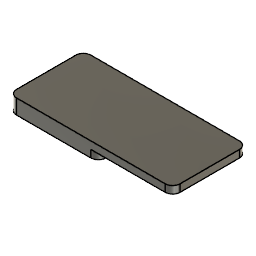
TAPAMESA (Autodesk Fusion 360 design; units mm, degrees)
part number: 2026-05-18-08-57-28-137
Autodesk Fusion 360 part; units mm, degrees
sketch "Sketch4" plane through (0, 0, 0) normal (0, 0, 1) x (1, 0, 0)
  line L0 (50, 0) -> (550, 0)
  line L1 (600, 50) -> (600, 450)
  line L2 (550, 500) -> (50, 500)
  line L3 (0, 450) -> (0, 50)
  arc A0 (600, 450) -> (550, 500) centre (550, 450) ccw
  arc A1 (550, 0) -> (600, 50) centre (550, 50) ccw
  arc A2 (50, 500) -> (0, 450) centre (50, 450) ccw
  arc A3 (0, 50) -> (50, 0) centre (50, 50) ccw
  line L4 (550, 500) -> (500, 500) construction
  line L5 (550, 0) -> (1050, 0)
  line L6 (1100, 50) -> (1100, 450)
  line L7 (1050, 500) -> (550, 500)
  arc A4 (1100, 450) -> (1050, 500) centre (1050, 450) ccw
  arc A5 (1050, 0) -> (1100, 50) centre (1050, 50) ccw
  point P0 (600, 0)
  point P1 (0, 500)
  point P2 (1100, 0)
  point P3 (1100, 0)
  point P4 (1100, 500)
  dimension "d20" = 600
  dimension "d21" = 500
  dimension "d22" = 50
  dimension "d23" = 50
  dimension "d24" = 50
  dimension "d25" = 50
  dimension "d42" = 550
  dimension "d43" = 500
  dimension "d44" = 50
  dimension "d45" = 50
  constraint horizontal L0
  constraint vertical L1
  constraint horizontal L2
  constraint vertical L3
  constraint tangent L1 A0
  constraint tangent L2 A0
  constraint coincident P0 L1
  constraint coincident P0 L0
  constraint tangent L1 A1
  constraint tangent L0 A1
  constraint coincident P1 L2
  constraint coincident P1 L3
  constraint tangent L2 A2
  constraint tangent L3 A2
  constraint coincident origin L0
  constraint coincident origin L3
  constraint tangent L0 A3
  constraint tangent L3 A3
  constraint coincident L2 L4.end
  constraint parallel L0 L5
  constraint perpendicular L0 L6
  constraint coincident P4 L6
  constraint coincident P4 L7
  constraint tangent L6 A4
  constraint tangent L7 A4
  constraint coincident P3 L5
  constraint coincident P3 L6
  constraint tangent L5 A5
  constraint tangent L6 A5
  measures "d20" distance of origin P0
  measures "d21" distance of origin P1
  measures "d22" radius of A0
  measures "d23" radius of A1
  measures "d24" radius of A2
  measures "d25" radius of A3
  measures "d42" distance of L0.end P3
  measures "d43" distance of P3 P4
  measures "d44" radius of A4
  measures "d45" radius of A5
extrude "Extrude7" add sketch "Sketch4" against normal blind 100 contours L0 L1 L2 L3 A0 A1 A2 A3
extrude "Extrude8" add sketch "Sketch4" against normal blind 50
